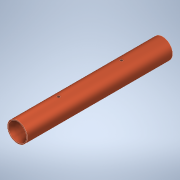
# Autodesk Inventor part: 4000_Cu_Bias_Shielding_(McMaster_50475K18)_MPSv2_v1
Saved by Autodesk Inventor 2021 (Build 250183000, 183)
## iProperties
Created: 2020-11-11
Part Number: 4000_Cu_Bias_Shielding_(McMaster_50475K18)_MPSv2_v1
Material: Copper
Document SubType Name: Modeling
Designer: Admin
Density: 8.94 g/cm^3
Appearance: Copper - Satin
Author: Admin
Autodesk Inventor part; units mm, degrees
ref_plane "YZ Plane" through (0, 0, 0) normal (1, 0, 0) x (0, 1, 0)
ref_plane "XZ Plane" through (0, 0, 0) normal (0, 1, 0) x (-1, 0, 0)
ref_plane "XY Plane" through (0, 0, 0) normal (0, 0, 1) x (1, 0, 0)
sketch "Sketch1" plane through (0, 0, 0) normal (0, 0, 1) x (1, 0, 0)
  circle A0 centre (0, 0) radius 18.8087
  circle A1 centre (0, 0) radius 20.6375
  dimension "d0" = 37.6174
  dimension "d1" = 41.275
  constraints: 2 centre point, 2 coincident
  measures "d0" diameter of A0
  measures "d1" diameter of A1
extrude "Extrusion1" add sketch "Sketch1" along normal blind 300
ref_plane "Work Plane1" through (-18.8087, 0, 0) normal (0, -1, 0) x (1, 0, 0)
sketch "Sketch3" plane through (-18.8087, 0, 0) normal (0, -1, 0) x (1, 0, 0)
  line L0 (18.8087, 0) -> (18.8087, 150)
  line L1 (18.8087, 0) -> (18.8087, 300) projected
  line L2 (18.8087, 150) -> (18.8087, 90)
  line L3 (18.8087, 90) -> (18.8087, 210)
  line L4 (18.8087, 90) -> (18.8087, 85)
  line L5 (18.8087, 210) -> (18.8087, 215)
  circle A0 centre (18.8087, 215) radius 2.5
  circle A1 centre (18.8087, 85) radius 2.5
  dimension "d6" = 150
  dimension "d7" = 60
  dimension "d8" = 120
  dimension "d9" = 5
  dimension "d10" = 5
  dimension "d11" = 5
  dimension "d12" = 5
  constraints: 10 end point, 4 point on line, 2 centre point, 2 coincident, 1 midpoint
  measures "d6" distance of L0.start L0.end
  measures "d7" distance of L0.end L2.end
  measures "d8" distance of L2.end L3.end
  measures "d9" distance of L2.end L4.end
  measures "d10" distance of L3.end L5.end
  measures "d11" diameter of A0
  measures "d12" diameter of A1
extrude "Extrusion3" cut sketch "Sketch3" along normal mid plane 300
body "Solid1"
